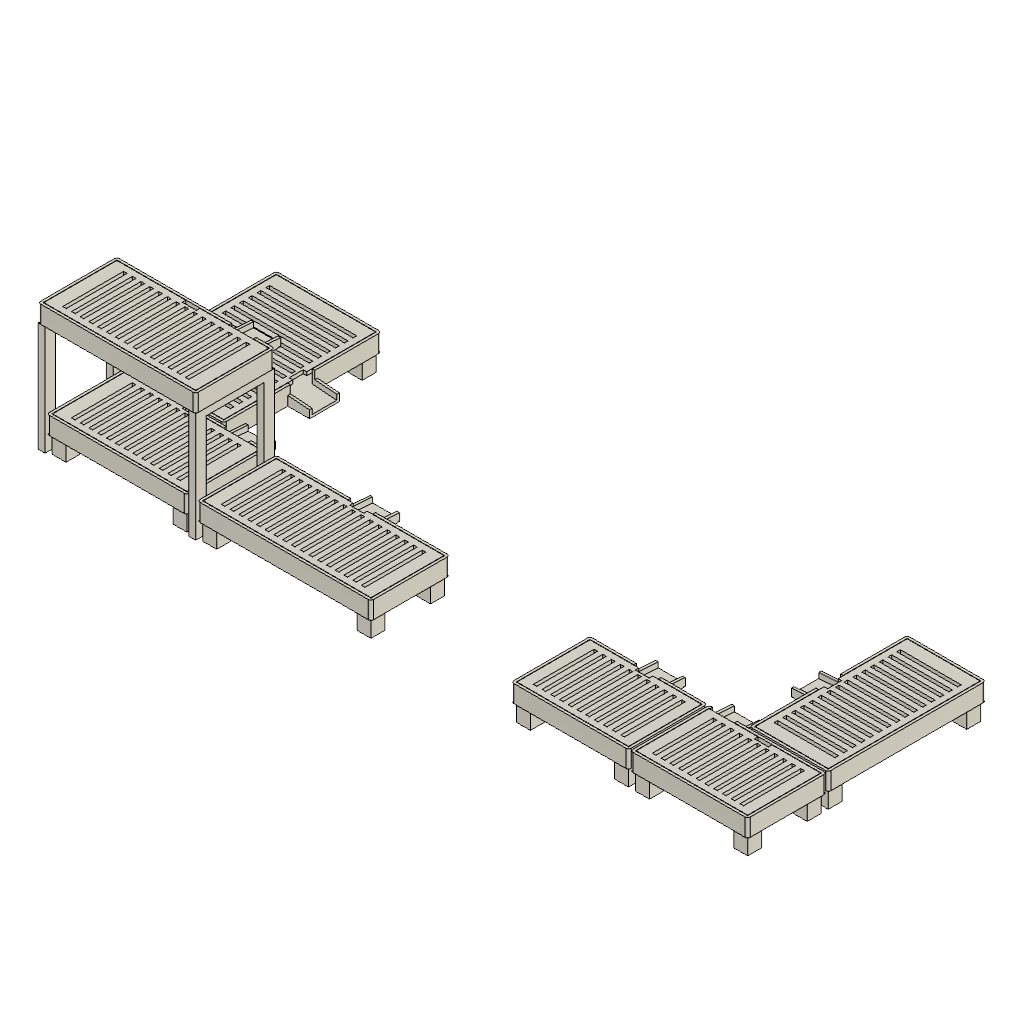
Sink_Organizer_B_R01_Prototype (Autodesk Fusion 360 design; units mm, degrees)
Autodesk Fusion 360 part; units mm, degrees
(part 1 of 8)
ref_plane "工作平面1" through (0, 0, 20) normal (0, 0, 1) x (1, 0, 0) in component "L1_DrainPan"
sketch "草图1" plane through (0, 0, 20) normal (0, 0, 1) x (1, 0, 0) in component "L1_DrainPan"
  line L0 (60, 50) -> (220, 50)
  line L1 (220, 50) -> (220, 140)
  line L2 (220, 140) -> (60, 140)
  line L3 (60, 140) -> (60, 50)
  dimension "d40" = 60
  dimension "d41" = 50
  dimension "d42" = 160
  dimension "d43" = 90
  constraint horizontal L0
  constraint vertical L1
  constraint horizontal L2
  constraint vertical L3
  measures "d40" horizontal distance of origin L0.start
  measures "d41" vertical distance of origin L0.start
  measures "d42" horizontal distance of L0.start L0.end
  measures "d43" vertical distance of L0.end L1.end
extrude "Pan blank" add sketch "草图1" along normal blind 20 makes body 1 in component "L1_DrainPan"
fillet "Outside corner rounds" radius 3 4 edges at (60, 140, 30) (220, 140, 30) (220, 50, 30) (60, 50, 30) on bodies 1 in component "L1_DrainPan"
ref_plane "工作平面2" through (63, 0, 0) normal (1, 0, 0) x (0, 1, 0) in component "L1_DrainPan"
sketch "草图2" plane through (63, 0, 0) normal (1, 0, 0) x (0, 0, -1) in component "L1_DrainPan"
  line L0 (-30.8318, 53) -> (-24.958, 137)
  line L1 (-24.958, 137) -> (-41, 137)
  line L2 (-41, 137) -> (-41, 53)
  line L3 (-41, 53) -> (-30.8318, 53)
  dimension "LeftAvailable" = 400
  dimension "RightAvailable" = 300
  dimension "RearAvailable" = 100
  dimension "LeftSideAvailable" = 130
  dimension "MirrorClearance" = 300
  dimension "RightSideAvailable" = 100
  dimension "LeftReach" = 180
  dimension "RightReach" = 180
  dimension "FaucetGap" = 160
  dimension "LeftRun" = 380
  dimension "RightRun" = 270
  dimension "Depth" = 90
  dimension "LeftSideDepth" = 120
  dimension "RightSideDepth" = 90
  dimension "ModuleGap" = 2
  dimension "TowerWidth" = 180
  dimension "TowerFrame" = 8
  dimension "TowerClearance" = 2
  dimension "FootHeight" = 20
  dimension "PanHeight" = 20
  dimension "FloorMin" = 3
  dimension "Wall" = 3
  dimension "DrainSlope" = 4
  dimension "DeckThick" = 4
  dimension "DeckClearance" = 0.3
  dimension "RimBorder" = 7
  dimension "SlotWidth" = 4
  dimension "SlotPitch" = 10
  dimension "DrainWidth" = 28
  dimension "DrainExtension" = 25
  dimension "UpperDeckHeight" = 145
  dimension "FootSize" = 16
  dimension "PegSize" = 8
  dimension "PegHeight" = 1.5
  dimension "FitClearance" = 0.25
  dimension "BaseX" = 50
  dimension "BaseY" = 50
  dimension "d50" = 30.8318
  dimension "d52" = 24.958
  dimension "d54" = 41
  constraint horizontal L1
  constraint vertical L2
  constraint horizontal L3
  measures "d50" horizontal distance of origin L0.start
  measures "d52" horizontal distance of origin L0.end
  measures "d54" horizontal distance of origin L1.end
extrude "Sloped catch cavity" cut sketch "草图2" along normal blind 154 bodies 1 in component "L1_DrainPan"
ref_plane "工作平面3" through (172, 0, 0) normal (1, 0, 0) x (0, 1, 0) in component "L1_DrainPan"
sketch "草图3" plane through (172, 0, 0) normal (1, 0, 0) x (0, 0, -1) in component "L1_DrainPan"
  line L0 (-20, 137) -> (-20, 165)
  line L1 (-20, 165) -> (-23, 165)
  line L2 (-23, 165) -> (-24.958, 137)
  line L3 (-24.958, 137) -> (-20, 137)
  dimension "d62" = 23
  dimension "d63" = 24.958
  constraint vertical L0
  constraint horizontal L1
  constraint horizontal L3
  measures "d62" horizontal distance of origin L1.end
  measures "d63" horizontal distance of origin L2.end
extrude "Drain tongue floor" add sketch "草图3" along normal blind 34 bodies 1 in component "L1_DrainPan"
ref_plane "工作平面4" through (172, 0, 0) normal (1, 0, 0) x (0, 1, 0) in component "L1_DrainPan"
sketch "草图4" plane through (172, 0, 0) normal (1, 0, 0) x (0, 0, -1) in component "L1_DrainPan"
  line L0 (-20, 137) -> (-20, 165)
  line L1 (-20, 165) -> (-29, 165)
  line L2 (-29, 165) -> (-30.958, 137)
  line L3 (-30.958, 137) -> (-20, 137)
  dimension "d71" = 29
  dimension "d72" = 30.958
  constraint vertical L0
  constraint horizontal L1
  constraint horizontal L3
  measures "d71" horizontal distance of origin L1.end
  measures "d72" horizontal distance of origin L2.end
extrude "Tongue side rail" add sketch "草图4" along normal blind 3 bodies 1 in component "L1_DrainPan"
ref_plane "工作平面5" through (203, 0, 0) normal (1, 0, 0) x (0, 1, 0) in component "L1_DrainPan"
sketch "草图5" plane through (203, 0, 0) normal (1, 0, 0) x (0, 0, -1) in component "L1_DrainPan"
  line L0 (-20, 137) -> (-20, 165)
  line L1 (-20, 165) -> (-29, 165)
  line L2 (-29, 165) -> (-30.958, 137)
  line L3 (-30.958, 137) -> (-20, 137)
  dimension "d80" = 29
  dimension "d81" = 30.958
  constraint vertical L0
  constraint horizontal L1
  constraint horizontal L3
  measures "d80" horizontal distance of origin L1.end
  measures "d81" horizontal distance of origin L2.end
extrude "Tongue side rail (1)" add sketch "草图5" along normal blind 3 bodies 1 in component "L1_DrainPan"
ref_plane "工作平面6" through (175, 0, 0) normal (1, 0, 0) x (0, 1, 0) in component "L1_DrainPan"
sketch "草图6" plane through (175, 0, 0) normal (1, 0, 0) x (0, 0, -1) in component "L1_DrainPan"
  line L0 (-24.958, 137) -> (-23, 165)
  line L1 (-23, 165) -> (-41, 165)
  line L2 (-41, 165) -> (-41, 137)
  line L3 (-41, 137) -> (-24.958, 137)
  dimension "d86" = 24.958
  dimension "d88" = 23
  dimension "d90" = 41
  constraint horizontal L1
  constraint vertical L2
  constraint horizontal L3
  measures "d86" horizontal distance of origin L0.start
  measures "d88" horizontal distance of origin L0.end
  measures "d90" horizontal distance of origin L1.end
extrude "Open drain mouth" cut sketch "草图6" along normal blind 28 bodies 1 in component "L1_DrainPan"
ref_plane "工作平面7" through (0, 0, 20) normal (0, 0, 1) x (1, 0, 0) in component "L1_DrainPan"
sketch "草图7" plane through (0, 0, 20) normal (0, 0, 1) x (1, 0, 0) in component "L1_DrainPan"
  line L0 (63, 53) -> (75, 53)
  line L1 (75, 53) -> (75, 65)
  line L2 (75, 65) -> (63, 65)
  line L3 (63, 65) -> (63, 53)
  dimension "d97" = 12
  dimension "d98" = 12
  constraint horizontal L0
  constraint vertical L1
  constraint horizontal L2
  constraint vertical L3
  measures "d97" horizontal distance of L0.start L0.end
  measures "d98" vertical distance of L0.end L1.end
extrude "Grate seat 00" add sketch "草图7" along normal blind 16 bodies 1 in component "L1_DrainPan"
ref_plane "工作平面8" through (0, 0, 20) normal (0, 0, 1) x (1, 0, 0) in component "L1_DrainPan"
sketch "草图8" plane through (0, 0, 20) normal (0, 0, 1) x (1, 0, 0) in component "L1_DrainPan"
  line L0 (63, 125) -> (75, 125)
  line L1 (75, 125) -> (75, 137)
  line L2 (75, 137) -> (63, 137)
  line L3 (63, 137) -> (63, 125)
  dimension "d104" = 125
  dimension "d105" = 12
  dimension "d106" = 12
  constraint horizontal L0
  constraint vertical L1
  constraint horizontal L2
  constraint vertical L3
  measures "d104" vertical distance of origin L0.start
  measures "d105" horizontal distance of L0.start L0.end
  measures "d106" vertical distance of L0.end L1.end
extrude "Grate seat 01" add sketch "草图8" along normal blind 16 bodies 1 in component "L1_DrainPan"
ref_plane "工作平面9" through (0, 0, 20) normal (0, 0, 1) x (1, 0, 0) in component "L1_DrainPan"
sketch "草图9" plane through (0, 0, 20) normal (0, 0, 1) x (1, 0, 0) in component "L1_DrainPan"
  line L0 (205, 53) -> (217, 53)
  line L1 (217, 53) -> (217, 65)
  line L2 (217, 65) -> (205, 65)
  line L3 (205, 65) -> (205, 53)
  dimension "d111" = 205
  dimension "d113" = 12
  dimension "d114" = 12
  constraint horizontal L0
  constraint vertical L1
  constraint horizontal L2
  constraint vertical L3
  measures "d111" horizontal distance of origin L0.start
  measures "d113" horizontal distance of L0.start L0.end
  measures "d114" vertical distance of L0.end L1.end
extrude "Grate seat 10" add sketch "草图9" along normal blind 16 bodies 1 in component "L1_DrainPan"
ref_plane "工作平面10" through (0, 0, 20) normal (0, 0, 1) x (1, 0, 0) in component "L1_DrainPan"
sketch "草图10" plane through (0, 0, 20) normal (0, 0, 1) x (1, 0, 0) in component "L1_DrainPan"
  line L0 (205, 125) -> (217, 125)
  line L1 (217, 125) -> (217, 137)
  line L2 (217, 137) -> (205, 137)
  line L3 (205, 137) -> (205, 125)
  dimension "d119" = 205
  dimension "d120" = 125
  dimension "d121" = 12
  dimension "d122" = 12
  constraint horizontal L0
  constraint vertical L1
  constraint horizontal L2
  constraint vertical L3
  measures "d119" horizontal distance of origin L0.start
  measures "d120" vertical distance of origin L0.start
  measures "d121" horizontal distance of L0.start L0.end
  measures "d122" vertical distance of L0.end L1.end
extrude "Grate seat 11" add sketch "草图10" along normal blind 16 bodies 1 in component "L1_DrainPan"
ref_plane "工作平面11" through (172, 0, 0) normal (1, 0, 0) x (0, 1, 0) in component "L1_DrainPan"
sketch "草图11" plane through (172, 0, 0) normal (1, 0, 0) x (0, 0, -1) in component "L1_DrainPan"
  line L0 (-19.8, 163) -> (-19.8, 164)
  line L1 (-19.8, 164) -> (-20.6, 164)
  line L2 (-20.6, 164) -> (-20.6, 163)
  line L3 (-20.6, 163) -> (-19.8, 163)
  dimension "d127" = 19.8
  dimension "d128" = 163
  dimension "d129" = 164
  dimension "d130" = 20.6
  constraint vertical L0
  constraint horizontal L1
  constraint vertical L2
  constraint horizontal L3
  measures "d127" horizontal distance of origin L0.start
  measures "d128" vertical distance of origin L0.start
  measures "d129" vertical distance of origin L0.end
  measures "d130" horizontal distance of origin L1.end
extrude "Drip break underside groove" cut sketch "草图11" along normal blind 34 bodies 1 in component "L1_DrainPan"
ref_plane "工作平面12" through (0, 0, 20) normal (0, 0, 1) x (1, 0, 0) in component "L1_DrainPan"
sketch "草图12" plane through (0, 0, 20) normal (0, 0, 1) x (1, 0, 0) in component "L1_DrainPan"
  line L0 (66.75, 56.75) -> (75.25, 56.75)
  line L1 (75.25, 56.75) -> (75.25, 65.25)
  line L2 (75.25, 65.25) -> (66.75, 65.25)
  line L3 (66.75, 65.25) -> (66.75, 56.75)
  dimension "d135" = 66.75
  dimension "d136" = 56.75
  dimension "d137" = 8.5
  dimension "d138" = 8.5
  constraint horizontal L0
  constraint vertical L1
  constraint horizontal L2
  constraint vertical L3
  measures "d135" horizontal distance of origin L0.start
  measures "d136" vertical distance of origin L0.start
  measures "d137" horizontal distance of L0.start L0.end
  measures "d138" vertical distance of L0.end L1.end
extrude "Foot socket 00" cut sketch "草图12" along normal blind 1.8 bodies 1 in component "L1_DrainPan"
ref_plane "工作平面13" through (0, 0, 20) normal (0, 0, 1) x (1, 0, 0) in component "L1_DrainPan"
sketch "草图13" plane through (0, 0, 20) normal (0, 0, 1) x (1, 0, 0) in component "L1_DrainPan"
  line L0 (66.75, 124.75) -> (75.25, 124.75)
  line L1 (75.25, 124.75) -> (75.25, 133.25)
  line L2 (75.25, 133.25) -> (66.75, 133.25)
  line L3 (66.75, 133.25) -> (66.75, 124.75)
  dimension "d143" = 66.75
  dimension "d144" = 124.75
  dimension "d145" = 8.5
  dimension "d146" = 8.5
  constraint horizontal L0
  constraint vertical L1
  constraint horizontal L2
  constraint vertical L3
  measures "d143" horizontal distance of origin L0.start
  measures "d144" vertical distance of origin L0.start
  measures "d145" horizontal distance of L0.start L0.end
  measures "d146" vertical distance of L0.end L1.end
extrude "Foot socket 01" cut sketch "草图13" along normal blind 1.8 bodies 1 in component "L1_DrainPan"
ref_plane "工作平面14" through (0, 0, 20) normal (0, 0, 1) x (1, 0, 0) in component "L1_DrainPan"
sketch "草图14" plane through (0, 0, 20) normal (0, 0, 1) x (1, 0, 0) in component "L1_DrainPan"
  line L0 (204.75, 56.75) -> (213.25, 56.75)
  line L1 (213.25, 56.75) -> (213.25, 65.25)
  line L2 (213.25, 65.25) -> (204.75, 65.25)
  line L3 (204.75, 65.25) -> (204.75, 56.75)
  dimension "d151" = 204.75
  dimension "d152" = 56.75
  dimension "d153" = 8.5
  dimension "d154" = 8.5
  constraint horizontal L0
  constraint vertical L1
  constraint horizontal L2
  constraint vertical L3
  measures "d151" horizontal distance of origin L0.start
  measures "d152" vertical distance of origin L0.start
  measures "d153" horizontal distance of L0.start L0.end
  measures "d154" vertical distance of L0.end L1.end
extrude "Foot socket 10" cut sketch "草图14" along normal blind 1.8 bodies 1 in component "L1_DrainPan"
ref_plane "工作平面15" through (0, 0, 20) normal (0, 0, 1) x (1, 0, 0) in component "L1_DrainPan"
sketch "草图15" plane through (0, 0, 20) normal (0, 0, 1) x (1, 0, 0) in component "L1_DrainPan"
  line L0 (204.75, 124.75) -> (213.25, 124.75)
  line L1 (213.25, 124.75) -> (213.25, 133.25)
  line L2 (213.25, 133.25) -> (204.75, 133.25)
  line L3 (204.75, 133.25) -> (204.75, 124.75)
  dimension "d159" = 204.75
  dimension "d160" = 124.75
  dimension "d161" = 8.5
  dimension "d162" = 8.5
  constraint horizontal L0
  constraint vertical L1
  constraint horizontal L2
  constraint vertical L3
  measures "d159" horizontal distance of origin L0.start
  measures "d160" vertical distance of origin L0.start
  measures "d161" horizontal distance of L0.start L0.end
  measures "d162" vertical distance of L0.end L1.end
extrude "Foot socket 11" cut sketch "草图15" along normal blind 1.8 bodies 1 in component "L1_DrainPan"
ref_plane "工作平面1" through (0, 0, 36) normal (0, 0, 1) x (1, 0, 0) in component "L1_RemovableGrate"
sketch "草图1 (2)" plane through (0, 0, 36) normal (0, 0, 1) x (1, 0, 0) in component "L1_RemovableGrate"
  line L0 (63.3, 53.3) -> (216.7, 53.3)
  line L1 (216.7, 53.3) -> (216.7, 136.7)
  line L2 (216.7, 136.7) -> (63.3, 136.7)
  line L3 (63.3, 136.7) -> (63.3, 53.3)
  dimension "d169" = 153.4
  dimension "d170" = 83.4
  constraint horizontal L0
  constraint vertical L1
  constraint horizontal L2
  constraint vertical L3
  measures "d169" horizontal distance of L0.start L0.end
  measures "d170" vertical distance of L0.end L1.end
extrude "Horizontal removable deck" add sketch "草图1 (2)" along normal blind 4 separate body makes body 2 in component "L1_RemovableGrate"
ref_plane "工作平面2" through (0, 0, 36) normal (0, 0, 1) x (1, 0, 0) in component "L1_RemovableGrate"
sketch "草图2 (2)" plane through (0, 0, 36) normal (0, 0, 1) x (1, 0, 0) in component "L1_RemovableGrate"
  line L0 (78, 60.3) -> (82, 60.3)
  line L1 (82, 60.3) -> (82, 129.7)
  line L2 (82, 129.7) -> (78, 129.7)
  line L3 (78, 129.7) -> (78, 60.3)
  dimension "d175" = 78
  dimension "d177" = 4
  dimension "d178" = 69.4
  constraint horizontal L0
  constraint vertical L1
  constraint horizontal L2
  constraint vertical L3
  measures "d175" horizontal distance of origin L0.start
  measures "d177" horizontal distance of L0.start L0.end
  measures "d178" vertical distance of L0.end L1.end
extrude "Drain slot 1" cut sketch "草图2 (2)" along normal blind 4 bodies 2 in component "L1_RemovableGrate"
ref_plane "工作平面3" through (0, 0, 36) normal (0, 0, 1) x (1, 0, 0) in component "L1_RemovableGrate"
sketch "草图3 (2)" plane through (0, 0, 36) normal (0, 0, 1) x (1, 0, 0) in component "L1_RemovableGrate"
  line L0 (88, 60.3) -> (92, 60.3)
  line L1 (92, 60.3) -> (92, 129.7)
  line L2 (92, 129.7) -> (88, 129.7)
  line L3 (88, 129.7) -> (88, 60.3)
  dimension "d183" = 88
  dimension "d185" = 4
  dimension "d186" = 69.4
  constraint horizontal L0
  constraint vertical L1
  constraint horizontal L2
  constraint vertical L3
  measures "d183" horizontal distance of origin L0.start
  measures "d185" horizontal distance of L0.start L0.end
  measures "d186" vertical distance of L0.end L1.end
extrude "Drain slot 2" cut sketch "草图3 (2)" along normal blind 4 bodies 2 in component "L1_RemovableGrate"
ref_plane "工作平面4" through (0, 0, 36) normal (0, 0, 1) x (1, 0, 0) in component "L1_RemovableGrate"
sketch "草图4 (2)" plane through (0, 0, 36) normal (0, 0, 1) x (1, 0, 0) in component "L1_RemovableGrate"
  line L0 (98, 60.3) -> (102, 60.3)
  line L1 (102, 60.3) -> (102, 129.7)
  line L2 (102, 129.7) -> (98, 129.7)
  line L3 (98, 129.7) -> (98, 60.3)
  dimension "d191" = 98
  dimension "d193" = 4
  dimension "d194" = 69.4
  constraint horizontal L0
  constraint vertical L1
  constraint horizontal L2
  constraint vertical L3
  measures "d191" horizontal distance of origin L0.start
  measures "d193" horizontal distance of L0.start L0.end
  measures "d194" vertical distance of L0.end L1.end
extrude "Drain slot 3" cut sketch "草图4 (2)" along normal blind 4 bodies 2 in component "L1_RemovableGrate"
ref_plane "工作平面5" through (0, 0, 36) normal (0, 0, 1) x (1, 0, 0) in component "L1_RemovableGrate"
sketch "草图5 (2)" plane through (0, 0, 36) normal (0, 0, 1) x (1, 0, 0) in component "L1_RemovableGrate"
  line L0 (108, 60.3) -> (112, 60.3)
  line L1 (112, 60.3) -> (112, 129.7)
  line L2 (112, 129.7) -> (108, 129.7)
  line L3 (108, 129.7) -> (108, 60.3)
  dimension "d199" = 108
  dimension "d201" = 4
  dimension "d202" = 69.4
  constraint horizontal L0
  constraint vertical L1
  constraint horizontal L2
  constraint vertical L3
  measures "d199" horizontal distance of origin L0.start
  measures "d201" horizontal distance of L0.start L0.end
  measures "d202" vertical distance of L0.end L1.end
extrude "Drain slot 4" cut sketch "草图5 (2)" along normal blind 4 bodies 2 in component "L1_RemovableGrate"
ref_plane "工作平面6" through (0, 0, 36) normal (0, 0, 1) x (1, 0, 0) in component "L1_RemovableGrate"
sketch "草图6 (2)" plane through (0, 0, 36) normal (0, 0, 1) x (1, 0, 0) in component "L1_RemovableGrate"
  line L0 (118, 60.3) -> (122, 60.3)
  line L1 (122, 60.3) -> (122, 129.7)
  line L2 (122, 129.7) -> (118, 129.7)
  line L3 (118, 129.7) -> (118, 60.3)
  dimension "d207" = 118
  dimension "d209" = 4
  dimension "d210" = 69.4
  constraint horizontal L0
  constraint vertical L1
  constraint horizontal L2
  constraint vertical L3
  measures "d207" horizontal distance of origin L0.start
  measures "d209" horizontal distance of L0.start L0.end
  measures "d210" vertical distance of L0.end L1.end
extrude "Drain slot 5" cut sketch "草图6 (2)" along normal blind 4 bodies 2 in component "L1_RemovableGrate"
ref_plane "工作平面7" through (0, 0, 36) normal (0, 0, 1) x (1, 0, 0) in component "L1_RemovableGrate"
sketch "草图7 (2)" plane through (0, 0, 36) normal (0, 0, 1) x (1, 0, 0) in component "L1_RemovableGrate"
  line L0 (128, 60.3) -> (132, 60.3)
  line L1 (132, 60.3) -> (132, 129.7)
  line L2 (132, 129.7) -> (128, 129.7)
  line L3 (128, 129.7) -> (128, 60.3)
  dimension "d215" = 128
  dimension "d217" = 4
  dimension "d218" = 69.4
  constraint horizontal L0
  constraint vertical L1
  constraint horizontal L2
  constraint vertical L3
  measures "d215" horizontal distance of origin L0.start
  measures "d217" horizontal distance of L0.start L0.end
  measures "d218" vertical distance of L0.end L1.end
extrude "Drain slot 6" cut sketch "草图7 (2)" along normal blind 4 bodies 2 in component "L1_RemovableGrate"
ref_plane "工作平面8" through (0, 0, 36) normal (0, 0, 1) x (1, 0, 0) in component "L1_RemovableGrate"
sketch "草图8 (2)" plane through (0, 0, 36) normal (0, 0, 1) x (1, 0, 0) in component "L1_RemovableGrate"
  line L0 (138, 60.3) -> (142, 60.3)
  line L1 (142, 60.3) -> (142, 129.7)
  line L2 (142, 129.7) -> (138, 129.7)
  line L3 (138, 129.7) -> (138, 60.3)
  dimension "d223" = 138
  dimension "d225" = 4
  dimension "d226" = 69.4
  constraint horizontal L0
  constraint vertical L1
  constraint horizontal L2
  constraint vertical L3
  measures "d223" horizontal distance of origin L0.start
  measures "d225" horizontal distance of L0.start L0.end
  measures "d226" vertical distance of L0.end L1.end
extrude "Drain slot 7" cut sketch "草图8 (2)" along normal blind 4 bodies 2 in component "L1_RemovableGrate"
ref_plane "工作平面9" through (0, 0, 36) normal (0, 0, 1) x (1, 0, 0) in component "L1_RemovableGrate"
sketch "草图9 (2)" plane through (0, 0, 36) normal (0, 0, 1) x (1, 0, 0) in component "L1_RemovableGrate"
  line L0 (148, 60.3) -> (152, 60.3)
  line L1 (152, 60.3) -> (152, 129.7)
  line L2 (152, 129.7) -> (148, 129.7)
  line L3 (148, 129.7) -> (148, 60.3)
  dimension "d231" = 148
  dimension "d233" = 4
  dimension "d234" = 69.4
  constraint horizontal L0
  constraint vertical L1
  constraint horizontal L2
  constraint vertical L3
  measures "d231" horizontal distance of origin L0.start
  measures "d233" horizontal distance of L0.start L0.end
  measures "d234" vertical distance of L0.end L1.end
extrude "Drain slot 8" cut sketch "草图9 (2)" along normal blind 4 bodies 2 in component "L1_RemovableGrate"
ref_plane "工作平面10" through (0, 0, 36) normal (0, 0, 1) x (1, 0, 0) in component "L1_RemovableGrate"
sketch "草图10 (2)" plane through (0, 0, 36) normal (0, 0, 1) x (1, 0, 0) in component "L1_RemovableGrate"
  line L0 (158, 60.3) -> (162, 60.3)
  line L1 (162, 60.3) -> (162, 129.7)
  line L2 (162, 129.7) -> (158, 129.7)
  line L3 (158, 129.7) -> (158, 60.3)
  dimension "d239" = 158
  dimension "d241" = 4
  dimension "d242" = 69.4
  constraint horizontal L0
  constraint vertical L1
  constraint horizontal L2
  constraint vertical L3
  measures "d239" horizontal distance of origin L0.start
  measures "d241" horizontal distance of L0.start L0.end
  measures "d242" vertical distance of L0.end L1.end
extrude "Drain slot 9" cut sketch "草图10 (2)" along normal blind 4 bodies 2 in component "L1_RemovableGrate"
ref_plane "工作平面11" through (0, 0, 36) normal (0, 0, 1) x (1, 0, 0) in component "L1_RemovableGrate"
sketch "草图11 (2)" plane through (0, 0, 36) normal (0, 0, 1) x (1, 0, 0) in component "L1_RemovableGrate"
  line L0 (168, 60.3) -> (172, 60.3)
  line L1 (172, 60.3) -> (172, 129.7)
  line L2 (172, 129.7) -> (168, 129.7)
  line L3 (168, 129.7) -> (168, 60.3)
  dimension "d247" = 168
  dimension "d249" = 4
  dimension "d250" = 69.4
  constraint horizontal L0
  constraint vertical L1
  constraint horizontal L2
  constraint vertical L3
  measures "d247" horizontal distance of origin L0.start
  measures "d249" horizontal distance of L0.start L0.end
  measures "d250" vertical distance of L0.end L1.end
extrude "Drain slot 10" cut sketch "草图11 (2)" along normal blind 4 bodies 2 in component "L1_RemovableGrate"
ref_plane "工作平面12" through (0, 0, 36) normal (0, 0, 1) x (1, 0, 0) in component "L1_RemovableGrate"
sketch "草图12 (2)" plane through (0, 0, 36) normal (0, 0, 1) x (1, 0, 0) in component "L1_RemovableGrate"
  line L0 (178, 60.3) -> (182, 60.3)
  line L1 (182, 60.3) -> (182, 129.7)
  line L2 (182, 129.7) -> (178, 129.7)
  line L3 (178, 129.7) -> (178, 60.3)
  dimension "d255" = 178
  dimension "d257" = 4
  dimension "d258" = 69.4
  constraint horizontal L0
  constraint vertical L1
  constraint horizontal L2
  constraint vertical L3
  measures "d255" horizontal distance of origin L0.start
  measures "d257" horizontal distance of L0.start L0.end
  measures "d258" vertical distance of L0.end L1.end
extrude "Drain slot 11" cut sketch "草图12 (2)" along normal blind 4 bodies 2 in component "L1_RemovableGrate"
ref_plane "工作平面13" through (0, 0, 36) normal (0, 0, 1) x (1, 0, 0) in component "L1_RemovableGrate"
sketch "草图13 (2)" plane through (0, 0, 36) normal (0, 0, 1) x (1, 0, 0) in component "L1_RemovableGrate"
  line L0 (188, 60.3) -> (192, 60.3)
  line L1 (192, 60.3) -> (192, 129.7)
  line L2 (192, 129.7) -> (188, 129.7)
  line L3 (188, 129.7) -> (188, 60.3)
  dimension "d263" = 188
  dimension "d265" = 4
  dimension "d266" = 69.4
  constraint horizontal L0
  constraint vertical L1
  constraint horizontal L2
  constraint vertical L3
  measures "d263" horizontal distance of origin L0.start
  measures "d265" horizontal distance of L0.start L0.end
  measures "d266" vertical distance of L0.end L1.end
extrude "Drain slot 12" cut sketch "草图13 (2)" along normal blind 4 bodies 2 in component "L1_RemovableGrate"
ref_plane "工作平面14" through (0, 0, 36) normal (0, 0, 1) x (1, 0, 0) in component "L1_RemovableGrate"
sketch "草图14 (2)" plane through (0, 0, 36) normal (0, 0, 1) x (1, 0, 0) in component "L1_RemovableGrate"
  line L0 (198, 60.3) -> (202, 60.3)
  line L1 (202, 60.3) -> (202, 129.7)
  line L2 (202, 129.7) -> (198, 129.7)
  line L3 (198, 129.7) -> (198, 60.3)
  dimension "d271" = 198
  dimension "d273" = 4
  dimension "d274" = 69.4
  constraint horizontal L0
  constraint vertical L1
  constraint horizontal L2
  constraint vertical L3
  measures "d271" horizontal distance of origin L0.start
  measures "d273" horizontal distance of L0.start L0.end
  measures "d274" vertical distance of L0.end L1.end
extrude "Drain slot 13" cut sketch "草图14 (2)" along normal blind 4 bodies 2 in component "L1_RemovableGrate"
ref_plane "工作平面15" through (0, 0, 36) normal (0, 0, 1) x (1, 0, 0) in component "L1_RemovableGrate"
sketch "草图15 (2)" plane through (0, 0, 36) normal (0, 0, 1) x (1, 0, 0) in component "L1_RemovableGrate"
  line L0 (132, 132.7) -> (148, 132.7)
  line L1 (148, 132.7) -> (148, 137.7)
  line L2 (148, 137.7) -> (132, 137.7)
  line L3 (132, 137.7) -> (132, 132.7)
  dimension "d279" = 132
  dimension "d280" = 132.7
  dimension "d281" = 16
  dimension "d282" = 5
  constraint horizontal L0
  constraint vertical L1
  constraint horizontal L2
  constraint vertical L3
  measures "d279" horizontal distance of origin L0.start
  measures "d280" vertical distance of origin L0.start
  measures "d281" horizontal distance of L0.start L0.end
  measures "d282" vertical distance of L0.end L1.end
extrude "Finger lift notch" cut sketch "草图15 (2)" along normal blind 4 bodies 2 in component "L1_RemovableGrate"
ref_plane "工作平面1" through (0, 0, 0) normal (0, 0, 1) x (1, 0, 0) in component "L1_Foot_00"
sketch "草图1 (3)" plane through (0, 0, 0) normal (0, 0, 1) x (1, 0, 0) in component "L1_Foot_00"
  line L0 (63, 53) -> (79, 53)
  line L1 (79, 53) -> (79, 69)
  line L2 (79, 69) -> (63, 69)
  line L3 (63, 69) -> (63, 53)
  dimension "d287" = 63
  dimension "d288" = 53
  dimension "d289" = 16
  dimension "d290" = 16
  constraint horizontal L0
  constraint vertical L1
  constraint horizontal L2
  constraint vertical L3
  measures "d287" horizontal distance of origin L0.start
  measures "d288" vertical distance of origin L0.start
  measures "d289" horizontal distance of L0.start L0.end
  measures "d290" vertical distance of L0.end L1.end
extrude "Foot base" add sketch "草图1 (3)" along normal blind 20 separate body makes body 3 in component "L1_Foot_00"
ref_plane "工作平面2" through (0, 0, 20) normal (0, 0, 1) x (1, 0, 0) in component "L1_Foot_00"
sketch "草图2 (3)" plane through (0, 0, 20) normal (0, 0, 1) x (1, 0, 0) in component "L1_Foot_00"
  line L0 (67, 57) -> (75, 57)
  line L1 (75, 57) -> (75, 65)
  line L2 (75, 65) -> (67, 65)
  line L3 (67, 65) -> (67, 57)
  dimension "d295" = 67
  dimension "d296" = 57
  dimension "d297" = 8
  dimension "d298" = 8
  constraint horizontal L0
  constraint vertical L1
  constraint horizontal L2
  constraint vertical L3
  measures "d295" horizontal distance of origin L0.start
  measures "d296" vertical distance of origin L0.start
  measures "d297" horizontal distance of L0.start L0.end
  measures "d298" vertical distance of L0.end L1.end
extrude "Locating peg" add sketch "草图2 (3)" along normal blind 1.5 bodies 3 in component "L1_Foot_00"
ref_plane "工作平面1" through (0, 0, 0) normal (0, 0, 1) x (1, 0, 0) in component "L1_Foot_01"
sketch "草图1 (4)" plane through (0, 0, 0) normal (0, 0, 1) x (1, 0, 0) in component "L1_Foot_01"
  line L0 (63, 121) -> (79, 121)
  line L1 (79, 121) -> (79, 137)
  line L2 (79, 137) -> (63, 137)
  line L3 (63, 137) -> (63, 121)
  dimension "d303" = 63
  dimension "d304" = 121
  dimension "d305" = 16
  dimension "d306" = 16
  constraint horizontal L0
  constraint vertical L1
  constraint horizontal L2
  constraint vertical L3
  measures "d303" horizontal distance of origin L0.start
  measures "d304" vertical distance of origin L0.start
  measures "d305" horizontal distance of L0.start L0.end
  measures "d306" vertical distance of L0.end L1.end
extrude "Foot base'" add sketch "草图1 (4)" along normal blind 20 separate body makes body 4 in component "L1_Foot_01"
ref_plane "工作平面2" through (0, 0, 20) normal (0, 0, 1) x (1, 0, 0) in component "L1_Foot_01"
sketch "草图2 (4)" plane through (0, 0, 20) normal (0, 0, 1) x (1, 0, 0) in component "L1_Foot_01"
  line L0 (67, 125) -> (75, 125)
  line L1 (75, 125) -> (75, 133)
  line L2 (75, 133) -> (67, 133)
  line L3 (67, 133) -> (67, 125)
  dimension "d311" = 67
  dimension "d312" = 125
  dimension "d313" = 8
  dimension "d314" = 8
  constraint horizontal L0
  constraint vertical L1
  constraint horizontal L2
  constraint vertical L3
  measures "d311" horizontal distance of origin L0.start
  measures "d312" vertical distance of origin L0.start
  measures "d313" horizontal distance of L0.start L0.end
  measures "d314" vertical distance of L0.end L1.end
extrude "Locating peg'" add sketch "草图2 (4)" along normal blind 1.5 bodies 4 in component "L1_Foot_01"
ref_plane "工作平面1" through (0, 0, 0) normal (0, 0, 1) x (1, 0, 0) in component "L1_Foot_10"
sketch "草图1 (5)" plane through (0, 0, 0) normal (0, 0, 1) x (1, 0, 0) in component "L1_Foot_10"
  line L0 (201, 53) -> (217, 53)
  line L1 (217, 53) -> (217, 69)
  line L2 (217, 69) -> (201, 69)
  line L3 (201, 69) -> (201, 53)
  dimension "d319" = 201
  dimension "d320" = 53
  dimension "d321" = 16
  dimension "d322" = 16
  constraint horizontal L0
  constraint vertical L1
  constraint horizontal L2
  constraint vertical L3
  measures "d319" horizontal distance of origin L0.start
  measures "d320" vertical distance of origin L0.start
  measures "d321" horizontal distance of L0.start L0.end
  measures "d322" vertical distance of L0.end L1.end
extrude "Foot base''" add sketch "草图1 (5)" along normal blind 20 separate body makes body 5 in component "L1_Foot_10"
ref_plane "工作平面2" through (0, 0, 20) normal (0, 0, 1) x (1, 0, 0) in component "L1_Foot_10"
sketch "草图2 (5)" plane through (0, 0, 20) normal (0, 0, 1) x (1, 0, 0) in component "L1_Foot_10"
  line L0 (205, 57) -> (213, 57)
  line L1 (213, 57) -> (213, 65)
  line L2 (213, 65) -> (205, 65)
  line L3 (205, 65) -> (205, 57)
  dimension "d327" = 205
  dimension "d328" = 57
  dimension "d329" = 8
  dimension "d330" = 8
  constraint horizontal L0
  constraint vertical L1
  constraint horizontal L2
  constraint vertical L3
  measures "d327" horizontal distance of origin L0.start
  measures "d328" vertical distance of origin L0.start
  measures "d329" horizontal distance of L0.start L0.end
  measures "d330" vertical distance of L0.end L1.end
extrude "Locating peg''" add sketch "草图2 (5)" along normal blind 1.5 bodies 5 in component "L1_Foot_10"
ref_plane "工作平面1" through (0, 0, 0) normal (0, 0, 1) x (1, 0, 0) in component "L1_Foot_11"
sketch "草图1 (6)" plane through (0, 0, 0) normal (0, 0, 1) x (1, 0, 0) in component "L1_Foot_11"
  line L0 (201, 121) -> (217, 121)
  line L1 (217, 121) -> (217, 137)
  line L2 (217, 137) -> (201, 137)
  line L3 (201, 137) -> (201, 121)
  dimension "d335" = 201
  dimension "d336" = 121
  dimension "d337" = 16
  dimension "d338" = 16
  constraint horizontal L0
  constraint vertical L1
  constraint horizontal L2
  constraint vertical L3
  measures "d335" horizontal distance of origin L0.start
  measures "d336" vertical distance of origin L0.start
  measures "d337" horizontal distance of L0.start L0.end
  measures "d338" vertical distance of L0.end L1.end
extrude "Foot base'''" add sketch "草图1 (6)" along normal blind 20 separate body makes body 6 in component "L1_Foot_11"
ref_plane "工作平面2" through (0, 0, 20) normal (0, 0, 1) x (1, 0, 0) in component "L1_Foot_11"
sketch "草图2 (6)" plane through (0, 0, 20) normal (0, 0, 1) x (1, 0, 0) in component "L1_Foot_11"
  line L0 (205, 125) -> (213, 125)
  line L1 (213, 125) -> (213, 133)
  line L2 (213, 133) -> (205, 133)
  line L3 (205, 133) -> (205, 125)
  dimension "d343" = 205
  dimension "d344" = 125
  dimension "d345" = 8
  dimension "d346" = 8
  constraint horizontal L0
  constraint vertical L1
  constraint horizontal L2
  constraint vertical L3
  measures "d343" horizontal distance of origin L0.start
  measures "d344" vertical distance of origin L0.start
  measures "d345" horizontal distance of L0.start L0.end
  measures "d346" vertical distance of L0.end L1.end
extrude "Locating peg'''" add sketch "草图2 (6)" along normal blind 1.5 bodies 6 in component "L1_Foot_11"
ref_plane "工作平面1" through (0, 0, 20) normal (0, 0, 1) x (1, 0, 0) in component "L2_DrainPan"
sketch "草图1 (7)" plane through (0, 0, 20) normal (0, 0, 1) x (1, 0, 0) in component "L2_DrainPan"
  line L0 (232, 50) -> (430, 50)
  line L1 (430, 50) -> (430, 140)
  line L2 (430, 140) -> (232, 140)
  line L3 (232, 140) -> (232, 50)
  dimension "d351" = 232
  dimension "d352" = 50
  dimension "d353" = 198
  dimension "d354" = 90
  constraint horizontal L0
  constraint vertical L1
  constraint horizontal L2
  constraint vertical L3
  measures "d351" horizontal distance of origin L0.start
  measures "d352" vertical distance of origin L0.start
  measures "d353" horizontal distance of L0.start L0.end
  measures "d354" vertical distance of L0.end L1.end
extrude "Pan blank'" add sketch "草图1 (7)" along normal blind 20 separate body makes body 7 in component "L2_DrainPan"
fillet "Outside corner rounds'" radius 3 4 edges at (232, 140, 30) (430, 140, 30) (430, 50, 30) (232, 50, 30) on bodies 7 in component "L2_DrainPan"
ref_plane "工作平面2" through (235, 0, 0) normal (1, 0, 0) x (0, 1, 0) in component "L2_DrainPan"
sketch "草图2 (7)" plane through (235, 0, 0) normal (1, 0, 0) x (0, 0, -1) in component "L2_DrainPan"
  line L0 (-30.8318, 53) -> (-24.958, 137)
  line L1 (-24.958, 137) -> (-41, 137)
  line L2 (-41, 137) -> (-41, 53)
  line L3 (-41, 53) -> (-30.8318, 53)
  dimension "d361" = 30.8318
  dimension "d363" = 24.958
  dimension "d365" = 41
  constraint horizontal L1
  constraint vertical L2
  constraint horizontal L3
  measures "d361" horizontal distance of origin L0.start
  measures "d363" horizontal distance of origin L0.end
  measures "d365" horizontal distance of origin L1.end
extrude "Sloped catch cavity'" cut sketch "草图2 (7)" along normal blind 192 bodies 7 in component "L2_DrainPan"
ref_plane "工作平面3" through (314, 0, 0) normal (1, 0, 0) x (0, 1, 0) in component "L2_DrainPan"
sketch "草图3 (3)" plane through (314, 0, 0) normal (1, 0, 0) x (0, 0, -1) in component "L2_DrainPan"
  line L0 (-20, 137) -> (-20, 165)
  line L1 (-20, 165) -> (-23, 165)
  line L2 (-23, 165) -> (-24.958, 137)
  line L3 (-24.958, 137) -> (-20, 137)
  dimension "d373" = 23
  dimension "d374" = 24.958
  constraint vertical L0
  constraint horizontal L1
  constraint horizontal L3
  measures "d373" horizontal distance of origin L1.end
  measures "d374" horizontal distance of origin L2.end
extrude "Drain tongue floor'" add sketch "草图3 (3)" along normal blind 34 bodies 7 in component "L2_DrainPan"
ref_plane "工作平面4" through (314, 0, 0) normal (1, 0, 0) x (0, 1, 0) in component "L2_DrainPan"
sketch "草图4 (3)" plane through (314, 0, 0) normal (1, 0, 0) x (0, 0, -1) in component "L2_DrainPan"
  line L0 (-20, 137) -> (-20, 165)
  line L1 (-20, 165) -> (-29, 165)
  line L2 (-29, 165) -> (-30.958, 137)
  line L3 (-30.958, 137) -> (-20, 137)
  dimension "d382" = 29
  dimension "d383" = 30.958
  constraint vertical L0
  constraint horizontal L1
  constraint horizontal L3
  measures "d382" horizontal distance of origin L1.end
  measures "d383" horizontal distance of origin L2.end
extrude "Tongue side rail'" add sketch "草图4 (3)" along normal blind 3 bodies 7 in component "L2_DrainPan"
ref_plane "工作平面5" through (345, 0, 0) normal (1, 0, 0) x (0, 1, 0) in component "L2_DrainPan"
sketch "草图5 (3)" plane through (345, 0, 0) normal (1, 0, 0) x (0, 0, -1) in component "L2_DrainPan"
  line L0 (-20, 137) -> (-20, 165)
  line L1 (-20, 165) -> (-29, 165)
  line L2 (-29, 165) -> (-30.958, 137)
  line L3 (-30.958, 137) -> (-20, 137)
  dimension "d391" = 29
  dimension "d392" = 30.958
  constraint vertical L0
  constraint horizontal L1
  constraint horizontal L3
  measures "d391" horizontal distance of origin L1.end
  measures "d392" horizontal distance of origin L2.end
extrude "Tongue side rail (1)'" add sketch "草图5 (3)" along normal blind 3 bodies 7 in component "L2_DrainPan"
ref_plane "工作平面6" through (317, 0, 0) normal (1, 0, 0) x (0, 1, 0) in component "L2_DrainPan"
sketch "草图6 (3)" plane through (317, 0, 0) normal (1, 0, 0) x (0, 0, -1) in component "L2_DrainPan"
  line L0 (-24.958, 137) -> (-23, 165)
  line L1 (-23, 165) -> (-41, 165)
  line L2 (-41, 165) -> (-41, 137)
  line L3 (-41, 137) -> (-24.958, 137)
  dimension "d397" = 24.958
  dimension "d399" = 23
  dimension "d401" = 41
  constraint horizontal L1
  constraint vertical L2
  constraint horizontal L3
  measures "d397" horizontal distance of origin L0.start
  measures "d399" horizontal distance of origin L0.end
  measures "d401" horizontal distance of origin L1.end
extrude "Open drain mouth'" cut sketch "草图6 (3)" along normal blind 28 bodies 7 in component "L2_DrainPan"
ref_plane "工作平面7" through (0, 0, 20) normal (0, 0, 1) x (1, 0, 0) in component "L2_DrainPan"
sketch "草图7 (3)" plane through (0, 0, 20) normal (0, 0, 1) x (1, 0, 0) in component "L2_DrainPan"
  line L0 (235, 53) -> (247, 53)
  line L1 (247, 53) -> (247, 65)
  line L2 (247, 65) -> (235, 65)
  line L3 (235, 65) -> (235, 53)
  dimension "d408" = 12
  dimension "d409" = 12
  constraint horizontal L0
  constraint vertical L1
  constraint horizontal L2
  constraint vertical L3
  measures "d408" horizontal distance of L0.start L0.end
  measures "d409" vertical distance of L0.end L1.end
extrude "Grate seat 00'" add sketch "草图7 (3)" along normal blind 16 bodies 7 in component "L2_DrainPan"
ref_plane "工作平面8" through (0, 0, 20) normal (0, 0, 1) x (1, 0, 0) in component "L2_DrainPan"
sketch "草图8 (3)" plane through (0, 0, 20) normal (0, 0, 1) x (1, 0, 0) in component "L2_DrainPan"
  line L0 (235, 125) -> (247, 125)
  line L1 (247, 125) -> (247, 137)
  line L2 (247, 137) -> (235, 137)
  line L3 (235, 137) -> (235, 125)
  dimension "d415" = 125
  dimension "d416" = 12
  dimension "d417" = 12
  constraint horizontal L0
  constraint vertical L1
  constraint horizontal L2
  constraint vertical L3
  measures "d415" vertical distance of origin L0.start
  measures "d416" horizontal distance of L0.start L0.end
  measures "d417" vertical distance of L0.end L1.end
extrude "Grate seat 01'" add sketch "草图8 (3)" along normal blind 16 bodies 7 in component "L2_DrainPan"
ref_plane "工作平面9" through (0, 0, 20) normal (0, 0, 1) x (1, 0, 0) in component "L2_DrainPan"
sketch "草图9 (3)" plane through (0, 0, 20) normal (0, 0, 1) x (1, 0, 0) in component "L2_DrainPan"
  line L0 (415, 53) -> (427, 53)
  line L1 (427, 53) -> (427, 65)
  line L2 (427, 65) -> (415, 65)
  line L3 (415, 65) -> (415, 53)
  dimension "d422" = 415
  dimension "d424" = 12
  dimension "d425" = 12
  constraint horizontal L0
  constraint vertical L1
  constraint horizontal L2
  constraint vertical L3
  measures "d422" horizontal distance of origin L0.start
  measures "d424" horizontal distance of L0.start L0.end
  measures "d425" vertical distance of L0.end L1.end
extrude "Grate seat 10'" add sketch "草图9 (3)" along normal blind 16 bodies 7 in component "L2_DrainPan"
ref_plane "工作平面10" through (0, 0, 20) normal (0, 0, 1) x (1, 0, 0) in component "L2_DrainPan"
sketch "草图10 (3)" plane through (0, 0, 20) normal (0, 0, 1) x (1, 0, 0) in component "L2_DrainPan"
  line L0 (415, 125) -> (427, 125)
  line L1 (427, 125) -> (427, 137)
  line L2 (427, 137) -> (415, 137)
  line L3 (415, 137) -> (415, 125)
  dimension "d430" = 415
  dimension "d431" = 125
  dimension "d432" = 12
  dimension "d433" = 12
  constraint horizontal L0
  constraint vertical L1
  constraint horizontal L2
  constraint vertical L3
  measures "d430" horizontal distance of origin L0.start
  measures "d431" vertical distance of origin L0.start
  measures "d432" horizontal distance of L0.start L0.end
  measures "d433" vertical distance of L0.end L1.end
extrude "Grate seat 11'" add sketch "草图10 (3)" along normal blind 16 bodies 7 in component "L2_DrainPan"
ref_plane "工作平面11" through (314, 0, 0) normal (1, 0, 0) x (0, 1, 0) in component "L2_DrainPan"
sketch "草图11 (3)" plane through (314, 0, 0) normal (1, 0, 0) x (0, 0, -1) in component "L2_DrainPan"
  line L0 (-19.8, 163) -> (-19.8, 164)
  line L1 (-19.8, 164) -> (-20.6, 164)
  line L2 (-20.6, 164) -> (-20.6, 163)
  line L3 (-20.6, 163) -> (-19.8, 163)
  dimension "d438" = 19.8
  dimension "d439" = 163
  dimension "d440" = 164
  dimension "d441" = 20.6
  constraint vertical L0
  constraint horizontal L1
  constraint vertical L2
  constraint horizontal L3
  measures "d438" horizontal distance of origin L0.start
  measures "d439" vertical distance of origin L0.start
  measures "d440" vertical distance of origin L0.end
  measures "d441" horizontal distance of origin L1.end
extrude "Drip break underside groove'" cut sketch "草图11 (3)" along normal blind 34 bodies 7 in component "L2_DrainPan"
ref_plane "工作平面12" through (0, 0, 20) normal (0, 0, 1) x (1, 0, 0) in component "L2_DrainPan"
sketch "草图12 (3)" plane through (0, 0, 20) normal (0, 0, 1) x (1, 0, 0) in component "L2_DrainPan"
  line L0 (238.75, 56.75) -> (247.25, 56.75)
  line L1 (247.25, 56.75) -> (247.25, 65.25)
  line L2 (247.25, 65.25) -> (238.75, 65.25)
  line L3 (238.75, 65.25) -> (238.75, 56.75)
  dimension "d446" = 238.75
  dimension "d447" = 56.75
  dimension "d448" = 8.5
  dimension "d449" = 8.5
  constraint horizontal L0
  constraint vertical L1
  constraint horizontal L2
  constraint vertical L3
  measures "d446" horizontal distance of origin L0.start
  measures "d447" vertical distance of origin L0.start
  measures "d448" horizontal distance of L0.start L0.end
  measures "d449" vertical distance of L0.end L1.end
extrude "Foot socket 00'" cut sketch "草图12 (3)" along normal blind 1.8 bodies 7 in component "L2_DrainPan"
ref_plane "工作平面13" through (0, 0, 20) normal (0, 0, 1) x (1, 0, 0) in component "L2_DrainPan"
sketch "草图13 (3)" plane through (0, 0, 20) normal (0, 0, 1) x (1, 0, 0) in component "L2_DrainPan"
  line L0 (238.75, 124.75) -> (247.25, 124.75)
  line L1 (247.25, 124.75) -> (247.25, 133.25)
  line L2 (247.25, 133.25) -> (238.75, 133.25)
  line L3 (238.75, 133.25) -> (238.75, 124.75)
  dimension "d454" = 238.75
  dimension "d455" = 124.75
  dimension "d456" = 8.5
  dimension "d457" = 8.5
  constraint horizontal L0
  constraint vertical L1
  constraint horizontal L2
  constraint vertical L3
  measures "d454" horizontal distance of origin L0.start
  measures "d455" vertical distance of origin L0.start
  measures "d456" horizontal distance of L0.start L0.end
  measures "d457" vertical distance of L0.end L1.end
extrude "Foot socket 01'" cut sketch "草图13 (3)" along normal blind 1.8 bodies 7 in component "L2_DrainPan"
ref_plane "工作平面14" through (0, 0, 20) normal (0, 0, 1) x (1, 0, 0) in component "L2_DrainPan"
sketch "草图14 (3)" plane through (0, 0, 20) normal (0, 0, 1) x (1, 0, 0) in component "L2_DrainPan"
  line L0 (414.75, 56.75) -> (423.25, 56.75)
  line L1 (423.25, 56.75) -> (423.25, 65.25)
  line L2 (423.25, 65.25) -> (414.75, 65.25)
  line L3 (414.75, 65.25) -> (414.75, 56.75)
  dimension "d462" = 414.75
  dimension "d463" = 56.75
  dimension "d464" = 8.5
  dimension "d465" = 8.5
  constraint horizontal L0
  constraint vertical L1
  constraint horizontal L2
  constraint vertical L3
  measures "d462" horizontal distance of origin L0.start
  measures "d463" vertical distance of origin L0.start
  measures "d464" horizontal distance of L0.start L0.end
  measures "d465" vertical distance of L0.end L1.end
extrude "Foot socket 10'" cut sketch "草图14 (3)" along normal blind 1.8 bodies 7 in component "L2_DrainPan"
ref_plane "工作平面15" through (0, 0, 20) normal (0, 0, 1) x (1, 0, 0) in component "L2_DrainPan"
sketch "草图15 (3)" plane through (0, 0, 20) normal (0, 0, 1) x (1, 0, 0) in component "L2_DrainPan"
  line L0 (414.75, 124.75) -> (423.25, 124.75)
  line L1 (423.25, 124.75) -> (423.25, 133.25)
  line L2 (423.25, 133.25) -> (414.75, 133.25)
  line L3 (414.75, 133.25) -> (414.75, 124.75)
  dimension "d470" = 414.75
  dimension "d471" = 124.75
  dimension "d472" = 8.5
  dimension "d473" = 8.5
  constraint horizontal L0
  constraint vertical L1
  constraint horizontal L2
  constraint vertical L3
  measures "d470" horizontal distance of origin L0.start
  measures "d471" vertical distance of origin L0.start
  measures "d472" horizontal distance of L0.start L0.end
  measures "d473" vertical distance of L0.end L1.end
extrude "Foot socket 11'" cut sketch "草图15 (3)" along normal blind 1.8 bodies 7 in component "L2_DrainPan"
ref_plane "工作平面1" through (0, 0, 36) normal (0, 0, 1) x (1, 0, 0) in component "L2_RemovableGrate"
sketch "草图1 (8)" plane through (0, 0, 36) normal (0, 0, 1) x (1, 0, 0) in component "L2_RemovableGrate"
  line L0 (235.3, 53.3) -> (426.7, 53.3)
  line L1 (426.7, 53.3) -> (426.7, 136.7)
  line L2 (426.7, 136.7) -> (235.3, 136.7)
  line L3 (235.3, 136.7) -> (235.3, 53.3)
  dimension "d480" = 191.4
  dimension "d481" = 83.4
  constraint horizontal L0
  constraint vertical L1
  constraint horizontal L2
  constraint vertical L3
  measures "d480" horizontal distance of L0.start L0.end
  measures "d481" vertical distance of L0.end L1.end
extrude "Horizontal removable deck'" add sketch "草图1 (8)" along normal blind 4 separate body makes body 8 in component "L2_RemovableGrate"
ref_plane "工作平面2" through (0, 0, 36) normal (0, 0, 1) x (1, 0, 0) in component "L2_RemovableGrate"
sketch "草图2 (8)" plane through (0, 0, 36) normal (0, 0, 1) x (1, 0, 0) in component "L2_RemovableGrate"
  line L0 (249, 60.3) -> (253, 60.3)
  line L1 (253, 60.3) -> (253, 129.7)
  line L2 (253, 129.7) -> (249, 129.7)
  line L3 (249, 129.7) -> (249, 60.3)
  dimension "d486" = 249
  dimension "d488" = 4
  dimension "d489" = 69.4
  constraint horizontal L0
  constraint vertical L1
  constraint horizontal L2
  constraint vertical L3
  measures "d486" horizontal distance of origin L0.start
  measures "d488" horizontal distance of L0.start L0.end
  measures "d489" vertical distance of L0.end L1.end
extrude "Drain slot 1'" cut sketch "草图2 (8)" along normal blind 4 bodies 8 in component "L2_RemovableGrate"
ref_plane "工作平面3" through (0, 0, 36) normal (0, 0, 1) x (1, 0, 0) in component "L2_RemovableGrate"
sketch "草图3 (4)" plane through (0, 0, 36) normal (0, 0, 1) x (1, 0, 0) in component "L2_RemovableGrate"
  line L0 (259, 60.3) -> (263, 60.3)
  line L1 (263, 60.3) -> (263, 129.7)
  line L2 (263, 129.7) -> (259, 129.7)
  line L3 (259, 129.7) -> (259, 60.3)
  dimension "d494" = 259
  dimension "d496" = 4
  dimension "d497" = 69.4
  constraint horizontal L0
  constraint vertical L1
  constraint horizontal L2
  constraint vertical L3
  measures "d494" horizontal distance of origin L0.start
  measures "d496" horizontal distance of L0.start L0.end
  measures "d497" vertical distance of L0.end L1.end
extrude "Drain slot 2'" cut sketch "草图3 (4)" along normal blind 4 bodies 8 in component "L2_RemovableGrate"
ref_plane "工作平面4" through (0, 0, 36) normal (0, 0, 1) x (1, 0, 0) in component "L2_RemovableGrate"
sketch "草图4 (4)" plane through (0, 0, 36) normal (0, 0, 1) x (1, 0, 0) in component "L2_RemovableGrate"
  line L0 (269, 60.3) -> (273, 60.3)
  line L1 (273, 60.3) -> (273, 129.7)
  line L2 (273, 129.7) -> (269, 129.7)
  line L3 (269, 129.7) -> (269, 60.3)
  dimension "d502" = 269
  dimension "d504" = 4
  dimension "d505" = 69.4
  constraint horizontal L0
  constraint vertical L1
  constraint horizontal L2
  constraint vertical L3
  measures "d502" horizontal distance of origin L0.start
  measures "d504" horizontal distance of L0.start L0.end
  measures "d505" vertical distance of L0.end L1.end
extrude "Drain slot 3'" cut sketch "草图4 (4)" along normal blind 4 bodies 8 in component "L2_RemovableGrate"
ref_plane "工作平面5" through (0, 0, 36) normal (0, 0, 1) x (1, 0, 0) in component "L2_RemovableGrate"
sketch "草图5 (4)" plane through (0, 0, 36) normal (0, 0, 1) x (1, 0, 0) in component "L2_RemovableGrate"
  line L0 (279, 60.3) -> (283, 60.3)
  line L1 (283, 60.3) -> (283, 129.7)
  line L2 (283, 129.7) -> (279, 129.7)
  line L3 (279, 129.7) -> (279, 60.3)
  dimension "d510" = 279
  dimension "d512" = 4
  dimension "d513" = 69.4
  constraint horizontal L0
  constraint vertical L1
  constraint horizontal L2
  constraint vertical L3
  measures "d510" horizontal distance of origin L0.start
  measures "d512" horizontal distance of L0.start L0.end
  measures "d513" vertical distance of L0.end L1.end
extrude "Drain slot 4'" cut sketch "草图5 (4)" along normal blind 4 bodies 8 in component "L2_RemovableGrate"
ref_plane "工作平面6" through (0, 0, 36) normal (0, 0, 1) x (1, 0, 0) in component "L2_RemovableGrate"
sketch "草图6 (4)" plane through (0, 0, 36) normal (0, 0, 1) x (1, 0, 0) in component "L2_RemovableGrate"
  line L0 (289, 60.3) -> (293, 60.3)
  line L1 (293, 60.3) -> (293, 129.7)
  line L2 (293, 129.7) -> (289, 129.7)
  line L3 (289, 129.7) -> (289, 60.3)
  dimension "d518" = 289
  dimension "d520" = 4
  dimension "d521" = 69.4
  constraint horizontal L0
  constraint vertical L1
  constraint horizontal L2
  constraint vertical L3
  measures "d518" horizontal distance of origin L0.start
  measures "d520" horizontal distance of L0.start L0.end
  measures "d521" vertical distance of L0.end L1.end
extrude "Drain slot 5'" cut sketch "草图6 (4)" along normal blind 4 bodies 8 in component "L2_RemovableGrate"
ref_plane "工作平面7" through (0, 0, 36) normal (0, 0, 1) x (1, 0, 0) in component "L2_RemovableGrate"